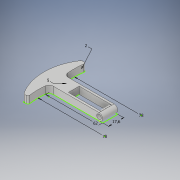
# Autodesk Inventor part: lever2
Saved by Autodesk Inventor 2019 (Build 230136000, 136)
## iProperties
Created: 2021-01-28
Part Number: lever2
Material: Genérico
Document SubType Name: Modeling
Designer: Juan M. Casillas
Density: 1 g/cm^3
Appearance: Valor por defecto
Author: Juan M. Casillas
Autodesk Inventor part; units mm, degrees
ref_plane "YZ Plane" through (0, 0, 0) normal (1, 0, 0) x (0, 1, 0)
ref_plane "XZ Plane" through (0, 0, 0) normal (0, 1, 0) x (-1, 0, 0)
ref_plane "XY Plane" through (0, 0, 0) normal (0, 0, 1) x (1, 0, 0)
sketch "Sketch1" plane through (0, 0, 0) normal (0, 1, 0) x (-1, 0, 0)
  circle A0 centre (45.6085, 8.8) radius 5.405
  line L0 (3.774, 0.6) -> (39.2972, 0.6)
  line L1 (3.774, 17) -> (3.774, 0.6)
  line L2 (39.2972, 17) -> (3.774, 17)
  line L3 (39.2972, 0.6) -> (39.2972, 17)
  arc A1 (64.4148, -24.0966) -> (64.4148, 41.6966) centre (14.2369, 8.8) ccw
  line L4 (61.1267, 42.6) -> (62.7422, 42.6)
  line L5 (5.5105, 17.6) -> (54.4325, 17.6)
  line L6 (54.4325, 0) -> (5.5105, 0)
  line L7 (62.7422, -25) -> (61.1267, -25)
  line L8 (-3.1893, 17.6) -> (-3.1893, 0)
  line L9 (54.4325, 0) -> (-3.1893, 0)
  line L10 (-3.1893, 17.6) -> (58.8107, 17.6)
  arc A2 (59.144, -22.7375) -> (59.406, -4.4863) centre (-18.1812, -12.5) ccw
  arc A3 (59.406, 22.0863) -> (59.144, 40.3375) centre (-18.1812, 30.1) ccw
  arc A4 (59.406, -4.4863) -> (54.4325, 0) centre (54.4325, -5) ccw
  arc A5 (54.4325, 17.6) -> (59.406, 22.0863) centre (54.4325, 22.6) ccw
  arc A6 (62.7422, -25) -> (64.4148, -24.0966) centre (62.7422, -23) ccw
  arc A7 (59.144, -22.7375) -> (61.1267, -25) centre (61.1267, -23) ccw
  arc A8 (61.1267, 42.6) -> (59.144, 40.3375) centre (61.1267, 40.6) ccw
  arc A9 (64.4148, 41.6966) -> (62.7422, 42.6) centre (62.7422, 40.6) ccw
  point P0 (0, 0)
  point P1 (17.5306, 8.8)
  point P2 (63.8107, -25)
  point P3 (63.8107, 42.6)
  dimension "d0" = 17.6
  dimension "d1" = 62
  dimension "d2" = 78
  dimension "d3" = 78
  dimension "d4" = 5
  dimension "d5" = 2
  constraints: 22 end point, 21 point on circle, 12 tangent, 10 centre point, 4 equal radius, 3 point on line
  measures "d0" distance of L8.start L9.end
  measures "d1" distance of L8.start L10.end
  measures "d2" radius of A2
  measures "d3" radius of A3
  measures "d4" radius of A4
  measures "d5" radius of A6
extrude "Extrusion1" add sketch "Sketch1" along normal blind 8.3 contours A0 | L1 L2 L3 L0 | A6 L7 A7 A2 A4 L6 L9 L8 L10 L5 A5 A3 A8 L4 A9 A1
sketch "Sketch2" plane through (-54.4325, 0, 17.6) normal (0, 0, 1) x (1, 0, 0)
  line L0 (0, 0) -> (57.6218, 0) construction
  line L1 (57.6218, 0) -> (57.6218, 8.3)
  line L2 (0, 8.3) -> (57.6218, 8.3)
  line L3 (0, 0) -> (0, 8.3) construction
  line L4 (57.6218, 0) -> (57.6218, 8.3) construction
  line L5 (57.6218, 4.15) -> (52.9259, 4.15) construction
  circle A0 centre (53.4718, 4.15) radius 4.15
  circle A1 centre (53.4718, 4.15) radius 2.6
  line L6 (0, 8.3) -> (57.6218, 8.3) projected
  line L7 (57.6218, 0) -> (57.6218, 8.3) construction
  line L8 (0, 0) -> (57.6218, 0) construction
  line L9 (53.4718, 8.3) -> (57.6218, 8.3)
  line L10 (57.6218, 0) -> (57.6218, 8.3)
  line L11 (53.4718, 0) -> (57.6218, 0)
  point P0 (54.4325, 0)
  dimension "d8" = 1.55
  constraints: 12 end point, 2 centre point, 2 collinear, 2 point on circle, 2 point on line, 1 horizontal, 1 midpoint, 1 perpendicular
  measures "d8" radial gap between concentric circles of A0 A1
extrude "Extrusion2" cut sketch "Sketch2" against normal through all
sketch "Sketch3" plane through (-54.4325, 0, 17.6) normal (0, 0, 1) x (1, 0, 0)
  circle A0 centre (53.4718, 4.15) radius 2.6 construction
  arc A1 (53.4718, 8.3) -> (53.4718, 0) centre (53.4718, 4.15) ccw construction
  circle A2 centre (53.4718, 4.15) radius 4.15
  point P0 (54.4325, 0)
  constraints: 1 centre point, 1 coincident, 1 concentric
extrude "Extrusion3" add sketch "Sketch3" against normal up to surface (17.6 mm away)
sketch "Sketch4" plane through (-54.4325, 0, 17.6) normal (0, 0, 1) x (1, 0, 0)
  circle A0 centre (53.4718, 4.15) radius 2.6 projected
  point P0 (54.4325, 0)
extrude "Extrusion4" cut sketch "Sketch4" against normal through all
sketch "Sketch5" plane through (-54.4325, 0, 17.6) normal (0, 0, 1) x (1, 0, 0)
  point P0 (54.4325, 0)
sketch "Sketch6" plane through (0, 0, 0) normal (0, -1, 0) x (1, 0, 0)
  line L0 (-39.2972, 17) -> (-3.774, 17) projected
  line L1 (-39.2972, 0.6) -> (-39.2972, 17) projected
  line L2 (-3.774, 0.6) -> (-39.2972, 0.6) projected
  line L3 (-3.774, 17) -> (-3.774, 0.6) projected
  line L4 (-54.4325, 17.6) -> (-0.9607, 17.6) construction
  line L5 (-29.8249, 17.6) -> (-29.8249, 15.1) construction
  line L6 (-3.774, 14.6) -> (-3.774, 3)
  line L7 (-39.2972, 3) -> (-39.2972, 14.6)
  line L8 (-25.5022, 0) -> (-25.5022, 2.5)
  line L9 (-3.5607, 17.6) -> (-3.5607, 0) construction
  line L10 (-3.5607, 7.6434) -> (-5.0607, 7.6434) construction
  line L11 (-39.2972, 15.1) -> (-5.0607, 15.1)
  line L12 (-5.0607, 15.1) -> (-5.0607, 2.5)
  line L13 (-5.0607, 2.5) -> (-39.2972, 2.5)
  line L14 (-39.2972, 2.5) -> (-39.2972, 15.1)
  point P0 (0, 0)
  dimension "d15" = 2.5
  dimension "d16" = 11.6
  dimension "d19" = 2.5
  dimension "d20" = 1.5
  constraints: 18 end point, 5 point on line, 3 parallel, 3 perpendicular, 1 horizontal
  measures "d15" distance of L5.start L5.end
  measures "d16" distance of L6.start L6.end
  measures "d19" distance of L8.start L8.end
  measures "d20" distance of L10.start L10.end
extrude "Extrusion5" cut sketch "Sketch6" against normal blind 8.3 contours L11 L12 L13 L1
fillet "Fillet1" radius 4 2 edges at (-5.0607, 0, 8.8) (-5.0607, 8.3, 8.8)
body "Solid1"
